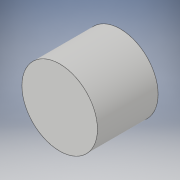
# Autodesk Inventor part: githubtestpart
Saved by Autodesk Inventor 2018.2 (Build 222227000, 227)
## iProperties
Created: 2018-04-26
Part Number: githubtestpart
Material: Generisch
Document SubType Name: Modeling
Designer: bened
Density: 1 g/cm^3
Appearance: Vorgabe
Author: bened
Autodesk Inventor part; units mm, degrees
ref_plane "YZ Plane" through (0, 0, 0) normal (1, 0, 0) x (0, 1, 0)
ref_plane "XZ Plane" through (0, 0, 0) normal (0, 1, 0) x (-1, 0, 0)
ref_plane "XY Plane" through (0, 0, 0) normal (0, 0, 1) x (1, 0, 0)
sketch "Sketch1" plane through (0, 0, 0) normal (0, 1, 0) x (-1, 0, 0)
  circle A0 centre (0.2839, 0) radius 6.2297
  point P0 (0, 0)
  dimension "d0" = 10
  constraints: 1 centre point
extrude "Extrusion1" add sketch "Sketch1" along normal blind 10
body "Solid1"
